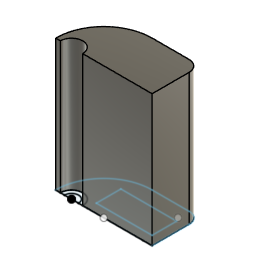
06 Antenna v4 (Autodesk Fusion 360 design; units mm, degrees)
Autodesk Fusion 360 part; units mm, degrees
sketch "antenna_nupsi" plane through (0, 0, 0) normal (0, 0, 1) x (1, 0, 0)
  line L0 (0, 0) -> (0.625, 0)
  line L1 (0.625, 0) -> (1.425, 0)
  line L2 (1.425, 0) -> (6.425, 0)
  line L3 (6.425, 0) -> (7.225, 0)
  line L4 (0, 0) -> (-0.625, 0)
  line L5 (-0.625, 0) -> (-1.425, 0)
  arc A0 (2.9, 4.325) -> (-1.425, 0) centre (2.9, 0) ccw
  line L6 (1.425, 0.8) -> (1.425, 3)
  line L7 (1.425, 3) -> (6.425, 3)
  line L8 (6.425, 3) -> (6.425, 0.8)
  line L9 (2.9, 4.325) -> (6.225, 4.325)
  line L10 (7.225, 0) -> (7.225, 3.325)
  line L11 (1.425, 0.8) -> (6.425, 0.8)
  arc A1 (0.625, 0) -> (-0.625, 0) centre (0, 0) ccw
  arc A2 (1, 0) -> (-1, 0) centre (0, 0) ccw
  arc A3 (7.225, 3.325) -> (6.225, 4.325) centre (6.225, 3.325) ccw
  dimension "d1" = 1.25
  dimension "d2" = 0.8
  dimension "d5" = 0.8
  dimension "d7" = 0.8
  dimension "d8" = 2.2
  dimension "d19" = 2
  dimension "d20" = 5
  constraint coincident L0.start L4.start
  constraint horizontal L0
  constraint parallel L0 L1
  constraint parallel L1 L2
  constraint parallel L2 L3
  constraint parallel L0 L4
  constraint parallel L4 L5
  constraint perpendicular L6 L7
  constraint tangent A0 L9
  constraint horizontal L9
  constraint tangent A0 L10
  constraint perpendicular L9 L10
  constraint perpendicular L8 L11
  constraint concentric A1 A2
  constraint coincident L5 A2.end
  constraint coincident L1 A2.start
  measures "d1" diameter of A1
  measures "d2" distance of L0.end L1.end
  measures "d5" distance of L4.end L5.end
  measures "d7" distance of L1.end L6.start
  measures "d8" distance of L6.start L6.end
  measures "d19" diameter of A2
  measures "d20" distance of L6.start L8.end
extrude "Extrude5" add sketch "antenna_nupsi" along normal blind 11 contours L1 L2 L3 L5 A0 L9 L10 A2 A3 makes body 1
extrude "Extrude6" add sketch "antenna_nupsi" along normal blind 0.8 separate body contours L1 L2 L3 L5 A0 L9 L10 A2 A3 | L6 L7 L8 L11 makes body 2
move_body "Move1" bodies 2 to x (1, 0, 0) y (0, 1, 0) z (0, 0, 1) at (0, 0, 11)
combine "Combine2" operation add target body 1 tool bodies 2
chamfer "Chamfer2" distance 0.25 angle 45 4 edges at (1.425, 1.9, 0) (3.925, 0.8, 0) (6.425, 1.9, 0) (3.925, 3, 0) on bodies 1
named bodies: "antenna_nupsi"
